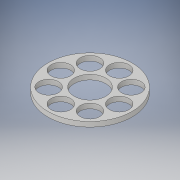
# Autodesk Inventor part: tubeholder
Saved by Autodesk Inventor 2019.3 (Build 233278000, 278)
## iProperties
Created: 2019-04-13
Part Number: tubeholder
Material: Generic
Document SubType Name: Modeling
Designer: peter
Density: 1 g/cm^3
Appearance: Default
Author: peter
Autodesk Inventor part; units mm, degrees
ref_plane "YZ Plane" through (0, 0, 0) normal (1, 0, 0) x (0, 1, 0)
ref_plane "XZ Plane" through (0, 0, 0) normal (0, 1, 0) x (-1, 0, 0)
ref_plane "XY Plane" through (0, 0, 0) normal (0, 0, 1) x (1, 0, 0)
sketch "Sketch1" plane through (0, 0, 0) normal (0, 1, 0) x (-1, 0, 0)
  line L0 (0, 0) -> (12, 0) construction
  circle A0 centre (12, 0) radius 4
  circle A1 centre (8.4853, 8.4853) radius 4
  circle A2 centre (0, 12) radius 4
  circle A3 centre (-8.4853, 8.4853) radius 4
  circle A4 centre (-12, 0) radius 4
  circle A5 centre (-8.4853, -8.4853) radius 4
  circle A6 centre (0, -12) radius 4
  circle A7 centre (8.4853, -8.4853) radius 4
  circle A8 centre (0, 0) radius 17.25
  circle A9 centre (0, 0) radius 6.5
  dimension "d0" = 12
  dimension "d1" = 8
  dimension "d4" = 360
  dimension "d6" = 34.5
  dimension "d9" = 13
  constraints: 10 centre point, 3 coincident, 2 end point, 1 horizontal, 17 other
  measures "d0" distance of L0.start L0.end
  measures "d1" diameter of A0
  measures "d6" diameter of A8
  measures "d9" diameter of A9
extrude "Extrusion1" add sketch "Sketch1" along normal blind 2
body "Solid1"
